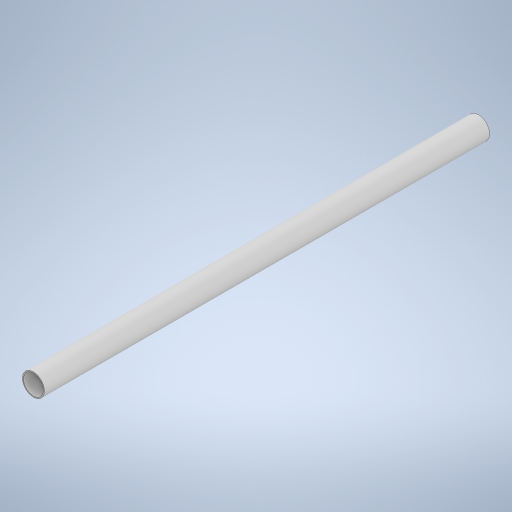
# Autodesk Inventor part: Round aluminium tube 20cm
Saved by Autodesk Inventor 2024 (Build 280153000, 153)
## iProperties
Created: 2023-09-10
Part Number: Round aluminium tube 20cm
Material: Generic
Document SubType Name: Modeling
Designer: AlfaNooraFithria
Density: 1 g/cm^3
Appearance: Default
Author: AlfaNooraFithria
Autodesk Inventor part; units mm, degrees
ref_plane "YZ Plane" through (0, 0, 0) normal (1, 0, 0) x (0, 1, 0)
ref_plane "XZ Plane" through (0, 0, 0) normal (0, 1, 0) x (-1, 0, 0)
ref_plane "XY Plane" through (0, 0, 0) normal (0, 0, 1) x (1, 0, 0)
sketch "Sketch1" plane through (0, 0, 0) normal (0, 0, 1) x (1, 0, 0)
  circle A0 centre (0, 0) radius 5
  dimension "d0" = 10
  constraints: 1 centre point, 1 coincident
  measures "d0" diameter of A0
extrude "Extrusion1" add sketch "Sketch1" against normal blind 200
shell "Shell1" thickness 0.5 removed faces 2 at (-0.591, 1.5584, 0) at (-0.591, 1.5584, -200)
body "Solid1"
